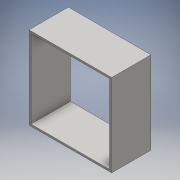
# Autodesk Inventor part: Part1
Saved by Autodesk Inventor 2016 (Build 200138000, 138)
## iProperties
Created: 2016-04-18
Part Number: Part1
Material: Generic
Document SubType Name: Modeling
Designer: Administrator
Density: 1 g/cm^3
Appearance: Default
Author: Administrator
Autodesk Inventor part; units mm, degrees
ref_plane "YZ Plane" through (0, 0, 0) normal (1, 0, 0) x (0, 1, 0)
ref_plane "XZ Plane" through (0, 0, 0) normal (0, 1, 0) x (-1, 0, 0)
ref_plane "XY Plane" through (0, 0, 0) normal (0, 0, 1) x (1, 0, 0)
sketch "Sketch1" plane through (0, 0, 0) normal (0, 1, 0) x (-1, 0, 0)
  line L0 (3.7114, 5.7847) -> (-16.2886, 5.7847)
  line L1 (-16.2886, 5.7847) -> (-16.2886, -14.2153)
  line L2 (-16.2886, -14.2153) -> (3.7114, -14.2153)
  line L3 (3.7114, -14.2153) -> (3.7114, 5.7847)
  line L4 (4.2114, 6.2847) -> (-16.7886, 6.2847)
  line L5 (-16.7886, 6.2847) -> (-16.7886, -14.7153)
  line L6 (-16.7886, -14.7153) -> (4.2114, -14.7153)
  line L7 (4.2114, -14.7153) -> (4.2114, 6.2847)
  point P0 (0, 0)
  dimension "d0" = 20
  dimension "d1" = 20
  dimension "d2" = 0.5
  constraints: 16 end point, 4 parallel, 2 perpendicular, 1 horizontal, 3 other
  measures "d0" distance of L2.end L1.end
  measures "d1" distance of L1.end L0.end
  measures "d2" distance between parallel lines of L3 L7
extrude "Extrusion2" add sketch "Sketch1" along normal blind 10
body "Solid2"
